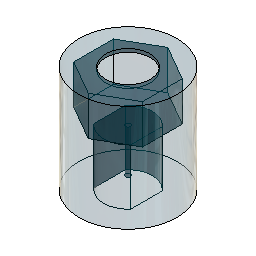
screw! v1 (Autodesk Fusion 360 design; units mm, degrees)
Autodesk Fusion 360 part; units mm, degrees
sketch "Sketch1" plane through (0, 0, 0) normal (0, 0, 1) x (1, 0, 0)
  line L0 (2.2449, -1.9139) -> (2.2449, 1.9139)
  arc A0 (2.2449, 1.9139) -> (-2.2449, 1.9139) centre (0, 0) ccw
  line L1 (-2.2449, 1.9139) -> (-2.2449, -1.9139)
  arc A1 (-2.2449, -1.9139) -> (2.2449, -1.9139) centre (0, 0) ccw
  circle A2 centre (0, 0) radius 0.3
sketch "Sketch2" plane through (0, 0, 0) normal (0, 0, 1) x (1, 0, 0)
  circle A0 centre (0, 0) radius 5.95
  dimension "d14" = 11.9
  measures "d14" diameter of A0
extrude "Extrude1" add sketch "Sketch2" along normal blind 13
extrude "Extrude2" cut sketch "Sketch1" along normal blind 6.8
sketch "Sketch3" plane through (0, 0, 13) normal (0, 0, 1) x (-1, 0, 0)
  circle A0 centre (0, 0) radius 5.95
  line L0 (4.2, -2.4249, -5.2) -> (4.2, 2.4249, -5.2)
  line L1 (4.2, 2.4249, -5.2) -> (0, 4.8497, -5.2)
  line L2 (0, 4.8497, -5.2) -> (-4.2, 2.4249, -5.2)
  line L3 (-4.2, 2.4249, -5.2) -> (-4.2, -2.4249, -5.2)
  line L4 (-4.2, -2.4249, -5.2) -> (0, -4.8497, -5.2)
  line L5 (0, -4.8497, -5.2) -> (4.2, -2.4249, -5.2)
  constraint coincident A0.centre origin
extrude "Extrude3" cut sketch "Sketch3" along normal blind 4.8 contours L0 L1 L2 L3 L4 L5 in plane through (0, 0, 7.8) normal (0, 0, 1)
sketch "Sketch4" plane through (0, 0, 13) normal (0, 0, 1) x (-1, 0, 0)
  circle A0 centre (0, 0) radius 5.95
  circle A1 centre (0, 0) radius 2.7
  dimension "d17" = 5.4
  constraint concentric A0 A1
  measures "d17" diameter of A1
extrude "Extrude4" cut sketch "Sketch4" against normal blind 1 contours A1
sketch "Sketch5" plane through (0, 0, 0) normal (0, 0, 1) x (1, 0, 0)
  circle A0 centre (0, 0) radius 0.5265
  constraint coincident A0.centre origin
extrude "Extrude5" cut sketch "Sketch5" along normal blind 1.5
equation "d8 = 7.8 mm + 5.2 mm"
